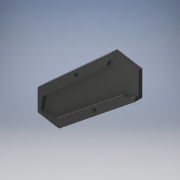
# Autodesk Inventor part: HA02
Saved by Autodesk Inventor 2017 (Build 210142000, 142)
## iProperties
Created: 2018-10-18
Part Number: HA02
Material: ABS Plastic
Document SubType Name: Modeling
Designer: Dell
Density: 1.06 g/cm^3
Appearance: Smooth - Black
Author: Dell
Autodesk Inventor part; units mm, degrees
ref_plane "XZ Plane" through (0, 0, 0) normal (0, 1, 0) x (-1, 0, 0)
ref_plane "XY Plane" through (0, 0, 0) normal (0, 0, 1) x (1, 0, 0)
sketch "Sketch1" plane through (0, 0, 0) normal (0, 0, 1) x (1, 0, 0)
  line L0 (0, 0) -> (100, 0)
  line L1 (100, 0) -> (100, 25)
  line L2 (100, 25) -> (0, 25)
  line L3 (0, 25) -> (0, 0)
  line L4 (0, 25) -> (115.2078, 140.2078)
  line L5 (100, 0) -> (177.7078, 77.7078)
  line L6 (151.2922, 176.2922) -> (200.5844, 163.0844)
  line L7 (200.5844, 163.0844) -> (213.7922, 113.7922)
  line L8 (213.7922, 113.7922) -> (177.7078, 77.7078)
  line L9 (177.7078, 77.7078) -> (128.4156, 90.9156)
  line L10 (128.4156, 90.9156) -> (115.2078, 140.2078)
  line L11 (115.2078, 140.2078) -> (151.2922, 176.2922)
  circle A0 centre (164.5, 127) radius 4
  dimension "d0" = 100
  dimension "d1" = 25
  dimension "d6" = 8
  dimension "d8" = 45
  dimension "d15" = 127
  constraints: 24 end point, 2 collinear, 2 parallel, 1 centre point, 1 coincident, 1 horizontal, 1 perpendicular, 13 other
  measures "d0" distance of L2.end L1.end
  measures "d1" distance of L1.end L0.end
  measures "d6" diameter of A0
  measures "d8" angle of L2 L4
  measures "d15" distance from line of L0 point (164.5, 127)
extrude "Extrusion1" add sketch "Sketch1" along normal blind 20
sketch "Sketch2" plane through (0, 0, 20) normal (0, 0, 1) x (1, 0, 0)
  line L0 (0, 25) -> (0, 0) projected
  line L1 (0, 0) -> (100, 0) projected
  line L2 (0, 25) -> (100, 25)
  line L3 (100, 25) -> (100, 0)
  line L4 (100, 0) -> (0, 0)
  line L5 (0, 0) -> (0, 25)
  line L6 (100, 25) -> (125, 25)
  line L7 (100, 0) -> (213.7922, 113.7922) projected
  line L8 (100, 0) -> (125, 25)
  constraints: 12 end point, 2 horizontal, 2 parallel, 1 perpendicular, 1 point on line
extrude "Extrusion2" add sketch "Sketch2" along normal blind 250
sketch "Sketch4" plane through (0, 0, 270) normal (0, 0, 1) x (1, 0, 0)
  line L0 (0, 25) -> (125, 25) projected
  line L1 (125, 25) -> (213.7922, 113.7922) projected
  line L2 (213.7922, 113.7922) -> (200.5844, 163.0844) projected
  line L3 (200.5844, 163.0844) -> (151.2922, 176.2922) projected
  line L4 (151.2922, 176.2922) -> (0, 25) projected
  circle A0 centre (164.5, 127) radius 4 projected
  line L5 (100, 0) -> (125, 25) projected
  line L6 (125, 25) -> (0, 25) projected
  line L7 (0, 25) -> (0, 0) projected
  line L8 (0, 0) -> (100, 0) projected
extrude "Extrusion3" add sketch "Sketch4" along normal blind 20
sketch "Sketch5" plane through (0, 0, 0) normal (0, -1, 0) x (1, 0, 0)
  line L0 (0, 0) -> (100, 0) projected
  line L1 (100, 0) -> (100, 290) projected
  line L2 (0, 290) -> (100, 290) projected
  line L3 (0, 0) -> (0, 290) projected
  line L4 (0, 0) -> (-125.5737, 72.5)
  line L5 (-125.5737, 72.5) -> (-125.5737, 217.5)
  line L6 (-125.5737, 217.5) -> (0, 290)
  line L7 (0, 290) -> (125.5737, 217.5)
  line L8 (125.5737, 217.5) -> (125.5737, 72.5)
  line L9 (125.5737, 72.5) -> (0, 0)
  point P0 (0, 145)
  constraints: 12 end point, 13 other
extrude "Extrusion4" add sketch "Sketch5" against normal blind 25 contours L4 L5 L6 L3
sketch "Sketch6" plane through (0, 25, 20) normal (0, 1, 0) x (1, 0, 0)
  line L0 (100, 20) -> (100, -270) projected
  circle A0 centre (-24.528, -125) radius 3
  circle A1 centre (-31.528, -125) radius 1.5
  circle A2 centre (-21.028, -131.0622) radius 1.5
  circle A3 centre (-21.028, -118.9378) radius 1.5
  point P0 (0, 20)
  point P1 (100, -125)
  dimension "d18" = 6
  dimension "d19" = 124.528
  dimension "d20" = 3
  dimension "d21" = 7
  dimension "d24" = 360
  constraints: 4 centre point, 2 horizontal alignment, 1 midpoint, 7 other
  measures "d18" diameter of A0
  measures "d19" distance from line of L0 A0.centre
  measures "d20" diameter of A1
  measures "d21" distance of A1.centre A0.centre
extrude "Extrusion5" cut sketch "Sketch6" against normal through all
sketch "Sketch7" plane through (100, 0, 0) normal (0, -1, 0) x (1, 0, 0)
  circle A0 centre (-124.528, 145) radius 3 projected
  circle A1 centre (-124.528, 145) radius 12
  point P0 (-100, 0)
  dimension "d28" = 24
  constraints: 1 centre point, 1 coincident
  measures "d28" diameter of A1
extrude "Extrusion6" cut sketch "Sketch7" against normal blind 5
sketch "Sketch8" plane through (0, 0, 270) normal (0, 0, -1) x (-1, 0, 0)
  circle A0 centre (-164.5, 127) radius 4 projected
  circle A1 centre (-164.5, 127) radius 12.5
  point P0 (0, 0)
  dimension "d31" = 25
  constraints: 1 centre point, 1 coincident
  measures "d31" diameter of A1
extrude "Extrusion7" cut sketch "Sketch8" against normal blind 7
sketch "Sketch10" plane through (164.5, 127, 277) normal (0, 0, -1) x (-1, 0, 0)
  circle A0 centre (7, 0) radius 2
  circle A1 centre (0, 0) radius 4 projected
  circle A2 centre (-3.5, 6.0622) radius 2
  circle A3 centre (-3.5, -6.0622) radius 2
  point P0 (164.5, -127)
  dimension "d34" = 4
  dimension "d37" = 360
  dimension "d39" = 7
  constraints: 3 centre point, 1 horizontal alignment, 7 other
  measures "d34" diameter of A0
  measures "d39" distance of A0.centre A1.centre
extrude "Extrusion8" cut sketch "Sketch10" against normal through all
sketch "Sketch11" plane through (0, 0, 290) normal (0, 0, 1) x (1, 0, 0)
  circle A0 centre (168, 133.0622) radius 2 projected
  circle A1 centre (164.5, 127) radius 4 projected
  circle A2 centre (168, 133.0622) radius 4
  circle A3 centre (157.5, 127) radius 4
  circle A4 centre (168, 120.9378) radius 4
  point P0 (0, 0)
  dimension "d42" = 8
  dimension "d45" = 360
  constraints: 3 centre point, 1 coincident, 7 other
  measures "d42" diameter of A2
extrude "Extrusion9" cut sketch "Sketch11" against normal blind 3 contours A0 | A1 A4 A3 A2 | A2 A1 | A1 A2 | A4 A1 | A1 A4 | A3 A1 | A1 A3
ref_plane "Work Plane1" through (164.5, 127, 270) normal (1, 0, 0) x (0, 0, 1)
sketch "Sketch12" plane through (164.5, 127, 270) normal (1, 0, 0) x (0, 0, 1)
  line L0 (17, -1.9365) -> (17, 1.9365) projected
  line L1 (17, 1.9365) -> (20, 1.9365) projected
  line L2 (20, 3.9993) -> (20, 1.9365) projected
  line L3 (20, 3.9993) -> (17, 3.9993) projected
  line L4 (17, 3.9993) -> (17, 2.0628) projected
  line L5 (17, 2.0628) -> (20, 2.0628) projected
  line L6 (20, -2.0628) -> (20, 2.0628) projected
  line L7 (20, -2.0628) -> (17, -2.0628) projected
  line L8 (17, -2.0628) -> (17, -3.9993) projected
  line L9 (17, -3.9993) -> (20, -3.9993) projected
  line L10 (20, -1.9365) -> (20, -3.9993) projected
  line L11 (20, -1.9365) -> (17, -1.9365) projected
  line L12 (7, 4) -> (7, -4) projected
  line L13 (7, -12.5) -> (7, 12.5) projected
  line L14 (0, -12.5) -> (0, 12.5) projected
  circle A0 centre (3.5, 0) radius 2
  line L15 (0, -12.5) -> (7, -12.5) projected
  point P0 (-270, 127)
  point P1 (7, 0)
  point P2 (3.5, -12.5)
  dimension "d50" = 4
  constraints: 2 midpoint, 1 centre point, 1 horizontal alignment, 1 vertical alignment
  measures "d50" diameter of A0
extrude "Extrusion10" cut sketch "Sketch12" along normal through all contours A0
sketch "Sketch13" plane through (0, 0, 20) normal (0, 0, 1) x (1, 0, 0)
  line L0 (100, 0) -> (213.7922, 113.7922) projected
  line L1 (213.7922, 113.7922) -> (200.5844, 163.0844) projected
  line L2 (200.5844, 163.0844) -> (151.2922, 176.2922) projected
  line L3 (151.2922, 176.2922) -> (0, 25) projected
  line L4 (0, 25) -> (0, 0) projected
  line L5 (0, 0) -> (100, 0) projected
  arc A0 (161, 128.9365) -> (161, 125.0635) centre (157.5, 127) ccw projected
  arc A1 (164.5729, 130.9993) -> (161, 128.9365) centre (164.5, 127) ccw projected
  arc A2 (167.9271, 129.0628) -> (164.5729, 130.9993) centre (168, 133.0622) ccw projected
  arc A3 (167.9271, 124.9372) -> (167.9271, 129.0628) centre (164.5, 127) ccw projected
  arc A4 (164.5729, 123.0007) -> (167.9271, 124.9372) centre (168, 120.9378) ccw projected
  arc A5 (161, 125.0635) -> (164.5729, 123.0007) centre (164.5, 127) ccw projected
  line L6 (-125.5737, 25) -> (0, 25) projected
  line L7 (0, 0) -> (-125.5737, 0) projected
  line L8 (0, 25) -> (0, 0) projected
  line L9 (-125.5737, 25) -> (0, 25) projected
  line L10 (-125.5737, 0) -> (-125.5737, 25) projected
extrude "Extrusion11" cut sketch "Sketch13" along normal through all contours L5 L4 L3 L2 L1 L0 | L7 L10 L6 L4 | A1 A2 A3 A4 A5 A0
sketch "Sketch14" plane through (0, 0, 20) normal (0, 0, 1) x (1, 0, 0)
  line L0 (-34.641, 0) -> (0, 0) projected
  line L1 (151.2922, 176.2922) -> (0, 25) projected
  line L2 (0, 0) -> (0, 25)
  line L3 (-34.641, 0) -> (-34.641, 25) projected
  line L4 (0, 25) -> (-34.641, 25)
  line L5 (-34.641, 25) -> (-34.641, 0)
  line L6 (-34.641, 0) -> (0, 0)
  constraints: 8 end point, 1 collinear, 1 perpendicular, 1 vertical
extrude "Extrusion12" cut sketch "Sketch14" against normal through all
sketch "Sketch15" plane through (0, 0, 20) normal (0, 0, 1) x (1, 0, 0)
  line L0 (15, 12.5) -> (90, 12.5) construction
  line L1 (0, 0) -> (100, 0) projected
  circle A0 centre (15, 12.5) radius 2.5
  circle A1 centre (90, 12.5) radius 2.5
  dimension "d57" = 75
  dimension "d58" = 12.5
  dimension "d59" = 10
  dimension "d60" = 5
  dimension "d61" = 5
  constraints: 2 centre point, 2 coincident, 2 end point, 1 horizontal
  measures "d57" distance of L0.start L0.end
  measures "d58" distance between parallel lines of L1 L0
  measures "d59" horizontal distance of L0.end L1.end
  measures "d60" diameter of A0
  measures "d61" diameter of A1
extrude "Extrusion13" cut sketch "Sketch15" against normal through all
sketch "Sketch16" plane through (0, 0, 20) normal (0, 0, 1) x (1, 0, 0)
  circle A0 centre (164.5, 127) radius 4 projected
  circle A1 centre (164.5, 127) radius 11.5
  point P0 (0, 0)
  dimension "d64" = 23
  constraints: 1 centre point, 1 coincident
  measures "d64" diameter of A1
extrude "Extrusion14" cut sketch "Sketch16" against normal through all
sketch "Sketch17" plane through (0, 0, 20) normal (0, 0, 1) x (1, 0, 0)
  circle A0 centre (164.5, 127) radius 11.5 projected
  circle A1 centre (164.5, 127) radius 22.5
  point P0 (0, 0)
  dimension "d67" = 45
  constraints: 1 centre point, 1 coincident
  measures "d67" diameter of A1
extrude "Extrusion15" cut sketch "Sketch17" against normal blind 10
sketch "Sketch18" plane through (0, 0, 20) normal (0, 0, 1) x (1, 0, 0)
  circle A0 centre (62.5, 40) radius 7.5
  line L0 (0, 25) -> (0, 0) projected
  line L1 (0, 25) -> (125, 25)
  line L2 (100, 0) -> (213.7922, 113.7922) projected
  point P0 (62.5, 25)
  dimension "d70" = 15
  dimension "d71" = 15
  constraints: 2 end point, 1 centre point, 1 horizontal, 1 midpoint, 1 point on line, 1 vertical alignment
  measures "d70" diameter of A0
  measures "d71" distance from line of A0.centre L1
extrude "Extrusion16" cut sketch "Sketch18" against normal through all
sketch "Sketch19" plane through (0, 0, 0) normal (0, 0, -1) x (-1, 0, 0)
  line L0 (-156.7794, 135.523) -> (-57.4648, 45.5585)
  circle A0 centre (-62.5, 40) radius 7.5 projected
  line L1 (-67.1947, 34.1511) -> (-171.6985, 118.0316)
  circle A1 centre (-164.5, 127) radius 11.5 projected
  circle A2 centre (-62.5, 40) radius 7.5 projected
  arc A3 (-156.7794, 135.523) -> (-171.6985, 118.0316) centre (-164.5, 127) ccw
  arc A4 (-67.1947, 34.1511) -> (-57.4648, 45.5585) centre (-62.5, 40) ccw
  point P0 (0, 0)
  constraints: 6 point on circle, 5 tangent, 4 end point, 2 centre point, 1 coincident, 4 other
extrude "Extrusion17" cut sketch "Sketch19" against normal blind 4
sketch "Sketch20" plane through (0, 0, 0) normal (0, 0, -1) x (-1, 0, 0)
  arc A0 (-156.7794, 135.523) -> (-171.6985, 118.0316) centre (-164.5, 127) ccw projected
  line L0 (-156.7794, 135.523) -> (-57.4648, 45.5585) projected
  line L1 (-67.1947, 34.1511) -> (-171.6985, 118.0316) projected
  arc A1 (-67.1947, 34.1511) -> (-57.4648, 45.5585) centre (-62.5, 40) ccw projected
  line L2 (-47.3944, 56.6755) -> (-146.709, 146.64)
  arc A2 (-146.709, 146.64) -> (-181.0879, 106.3338) centre (-164.5, 127) ccw
  line L3 (-181.0879, 106.3338) -> (-76.584, 22.4532)
  arc A3 (-76.584, 22.4532) -> (-47.3944, 56.6755) centre (-62.5, 40) ccw
  point P0 (0, 0)
  dimension "d76" = 15
  constraints: 4 end point, 4 point on circle, 2 centre point, 3 other
  measures "d76" distance between parallel lines of L0 L2
extrude "Extrusion18" cut sketch "Sketch20" against normal blind 5 contours L0 A1 L1 A0 | A3 L3 A2 L2
sketch "Sketch21" plane through (0, 0, 5) normal (0, 0, -1) x (-1, 0, 0)
  circle A0 centre (-62.5, 40) radius 7.5 projected
  circle A1 centre (-164.5, 127) radius 11.5 projected
  line L0 (-146.709, 146.64) -> (-47.3944, 56.6755) projected
  arc A2 (-146.709, 146.64) -> (-181.0879, 106.3338) centre (-164.5, 127) ccw projected
  line L1 (-76.584, 22.4532) -> (-181.0879, 106.3338) projected
  arc A3 (-76.584, 22.4532) -> (-47.3944, 56.6755) centre (-62.5, 40) ccw projected
  line L2 (-76.584, 22.4532) -> (-181.0879, 106.3338) projected
  line L3 (-128.8359, 64.3935) -> (-97.0517, 101.6578) construction
  line L4 (-146.709, 146.64) -> (-47.3944, 56.6755) projected
  circle A4 centre (-125.5912, 68.1977) radius 2.5
  circle A5 centre (-100.2965, 97.8536) radius 2.5
  point P0 (0, 0)
  dimension "d79" = 5
  dimension "d80" = 5
  dimension "d81" = 5
  dimension "d82" = 5
  constraints: 2 centre point, 2 end point, 2 midpoint, 2 point on line
  measures "d79" diameter of A4
  measures "d80" diameter of A5
  measures "d81" distance of L3.end A5.centre
  measures "d82" distance of L3.start A4.centre
extrude "Extrusion19" cut sketch "Sketch21" against normal through all contours A4 | A5
sketch "Sketch22" plane through (0, 0, 5) normal (0, 0, -1) x (-1, 0, 0)
  circle A0 centre (-125.5912, 68.1977) radius 2.5 projected
  circle A1 centre (-100.2965, 97.8536) radius 2.5 projected
  circle A2 centre (-62.5, 40) radius 7.5 projected
  circle A3 centre (-164.5, 127) radius 11.5 projected
  line L0 (-146.709, 146.64) -> (-47.3944, 56.6755) projected
  arc A4 (-146.709, 146.64) -> (-181.0879, 106.3338) centre (-164.5, 127) ccw projected
  line L1 (-76.584, 22.4532) -> (-181.0879, 106.3338) projected
  arc A5 (-76.584, 22.4532) -> (-47.3944, 56.6755) centre (-62.5, 40) ccw projected
  arc A6 (-146.709, 146.64) -> (-181.0879, 106.3338) centre (-164.5, 127) ccw projected
  line L2 (-146.709, 146.64) -> (-47.3944, 56.6755) projected
  arc A7 (-76.584, 22.4532) -> (-47.3944, 56.6755) centre (-62.5, 40) ccw projected
  line L3 (-76.584, 22.4532) -> (-181.0879, 106.3338) projected
  line L4 (0, 0) -> (-100, 0) projected
  line L5 (0, 25) -> (0, 0) projected
  line L6 (-151.2922, 176.2922) -> (0, 25) projected
  line L7 (-200.5844, 163.0844) -> (-151.2922, 176.2922) projected
  line L8 (-213.7922, 113.7922) -> (-200.5844, 163.0844) projected
  line L9 (-100, 0) -> (-213.7922, 113.7922) projected
  circle A8 centre (-90, 12.5) radius 2.5 projected
  circle A9 centre (-15, 12.5) radius 2.5 projected
extrude "Extrusion20" cut sketch "Sketch22" along normal through all both and the other way through all contours L4 L9 L8 L7 L6 L5
sketch "Sketch23" plane through (0, 0, 20) normal (0, 0, 1) x (1, 0, 0)
  line L0 (76.584, 22.4532) -> (181.0879, 106.3338) projected
  arc A0 (47.3944, 56.6755) -> (76.584, 22.4532) centre (62.5, 40) ccw projected
  line L1 (76.584, 22.4532) -> (181.0879, 106.3338) projected
  arc A1 (181.0879, 106.3338) -> (146.709, 146.64) centre (164.5, 127) ccw projected
  line L2 (146.709, 146.64) -> (47.3944, 56.6755) projected
  circle A2 centre (125.5912, 68.1977) radius 2.5 projected
  circle A3 centre (100.2965, 97.8536) radius 2.5 projected
  circle A4 centre (62.5, 40) radius 7.5 projected
  circle A5 centre (164.5, 127) radius 22.5 projected
  arc A6 (174.8283, 114.1323) -> (153.4226, 139.2287) centre (164.5, 127) ccw
  line L3 (174.8283, 114.1323) -> (70.3245, 30.2518)
  arc A7 (54.108, 49.2642) -> (70.3245, 30.2518) centre (62.5, 40) ccw
  line L4 (54.108, 49.2642) -> (153.4226, 139.2287)
  point P0 (0, 0)
  dimension "d87" = 10
  constraints: 4 end point, 4 point on circle, 2 centre point, 3 other
  measures "d87" radial gap between concentric circles of A1 A6
extrude "Extrusion21" cut sketch "Sketch23" against normal blind 10 contours L4 A6 L3 A5 | A5 L3 A7 L4 picked at (159.1311, 121.3058)
sketch "Sketch24" plane through (0, 0, 10) normal (0, 0, 1) x (1, 0, 0)
  circle A0 centre (62.5, 40) radius 7.5 projected
  circle A1 centre (164.5, 127) radius 11.5 projected
  point P0 (0, 0)
extrude "Extrusion22" add sketch "Sketch24" against normal blind 5
sketch "Sketch25" plane through (0, 0, 20) normal (0, 0, 1) x (1, 0, 0)
  line L0 (54.108, 49.2642) -> (142.0854, 128.9589) projected
  arc A0 (162.8988, 104.557) -> (142.0854, 128.9589) centre (164.5, 127) ccw projected
  line L1 (162.8988, 104.557) -> (70.3245, 30.2518) projected
  arc A1 (54.108, 49.2642) -> (70.3245, 30.2518) centre (62.5, 40) ccw projected
  arc A2 (47.3944, 56.6755) -> (76.584, 22.4532) centre (62.5, 40) ccw projected
  line L2 (76.584, 22.4532) -> (181.0879, 106.3338) projected
  arc A3 (181.0879, 106.3338) -> (146.709, 146.64) centre (164.5, 127) ccw projected
  line L3 (146.709, 146.64) -> (47.3944, 56.6755) projected
  circle A4 centre (125.5912, 68.1977) radius 2.5 projected
  circle A5 centre (100.2965, 97.8536) radius 2.5 projected
  point P0 (0, 0)
extrude "Extrusion23" cut sketch "Sketch25" against normal blind 5
sketch "Sketch26" plane through (0, 0, 5) normal (0, 0, -1) x (-1, 0, 0)
  arc A0 (-146.709, 146.64) -> (-181.0879, 106.3338) centre (-164.5, 127) ccw projected
  line L0 (-164.5, 127) -> (-180.8089, 140.9105)
  arc A1 (-76.584, 22.4532) -> (-47.3944, 56.6755) centre (-62.5, 40) ccw projected
  line L1 (-164.5, 127) -> (-62.5, 40)
  line L2 (-181.0879, 106.3338) -> (-180.8089, 140.9105)
  line L3 (-180.8089, 140.9105) -> (-146.709, 146.64)
  point P0 (0, 0)
  dimension "d95" = 100
  constraints: 8 end point, 1 collinear
  measures "d95" angle of L3 L2
extrude "Extrusion24" cut sketch "Sketch26" against normal through all
sketch "Sketch27" plane through (0, 0, 5) normal (0, 0, -1) x (-1, 0, 0)
  arc A0 (-76.584, 22.4532) -> (-47.3944, 56.6755) centre (-62.5, 40) ccw projected
  line L0 (-76.584, 22.4532) -> (-76.584, 22.4532)
  line L1 (-181.0879, 106.3338) -> (-76.584, 22.4532) projected
  arc A1 (-76.584, 22.4532) -> (-47.3944, 56.6755) centre (-62.5, 40) ccw projected
  line L2 (-76.584, 22.4532) -> (-47.3944, 56.6755)
  point P0 (0, 0)
  constraints: 4 end point
extrude "Extrusion25" cut sketch "Sketch27" against normal through all
sketch "Sketch28" plane through (0, 0, 5) normal (0, 0, -1) x (-1, 0, 0)
  line L0 (-76.584, 22.4532) -> (-47.3944, 56.6755) projected
  line L1 (-76.584, 22.4532) -> (-47.6313, 27.3179)
  line L2 (-47.6313, 27.3179) -> (-47.3944, 56.6755)
  line L3 (-180.8089, 140.9105) -> (-47.6313, 27.3179)
  point P0 (0, 0)
  point P1 (-61.9892, 39.5643)
  dimension "d101" = 100
  constraints: 6 end point, 1 midpoint, 1 point on line
  measures "d101" angle of L2 L1
extrude "Extrusion26" add sketch "Sketch28" against normal blind 10
sketch "Sketch30" plane through (0, 0, 15) normal (0, 0, 1) x (1, 0, 0)
  line L0 (70.0894, 30.0676) -> (53.8891, 49.061) projected
  line L1 (53.8891, 49.061) -> (51.4355, 30.5626)
  line L2 (51.4355, 30.5626) -> (70.0894, 30.0676)
  line L3 (76.584, 22.4532) -> (47.6313, 27.3179) projected
  line L4 (47.6313, 27.3179) -> (61.9892, 39.5643)
  point P0 (0, 0)
  dimension "d105" = 5
  constraints: 6 end point, 1 midpoint, 1 perpendicular, 1 point on line
  measures "d105" distance of L3.end L1.end
extrude "Extrusion27" cut sketch "Sketch30" against normal blind 5
body "Solid1"
